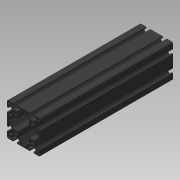
# Autodesk Inventor part: 3030-LS
Saved by Autodesk Inventor 2013 (Build 170138000, 138)
## iProperties
Company: 80/20 Inc.
Created: 2014-04-23
Part Number: 3030-LS
Material: Generic
Document SubType Name: Modeling
Density: 1 g/cm^3
Vendor: 80/20 Inc.
Engineer: Ross Bowman
Designer: Ross Bowman
Catalog Web Link: 8020.net
Material: 6105-T5 Aluminum
Author: Ross Bowman
Keywords: 80/20 , 8020 , T-Slot , Extrusion
Autodesk Inventor part; units mm, degrees
ref_plane "YZ Plane" through (0, 0, 0) normal (1, 0, 0) x (0, 1, 0)
ref_plane "XZ Plane" through (0, 0, 0) normal (0, 1, 0) x (-1, 0, 0)
ref_plane "XY Plane" through (0, 0, 0) normal (0, 0, 1) x (1, 0, 0)
sketch "Sketch1" plane through (0, 0, 0) normal (0, 0, 1) x (1, 0, 0)
  arc A0 (14.8044, -21.6898) -> (16.4102, -23.2956) centre (15.5149, -22.5851) ccw
  line L0 (16.0771, -20.4064) -> (14.8044, -21.6898)
  arc A1 (16.0771, -17.6936) -> (16.0771, -20.4064) centre (19.05, -19.05) ccw
  line L1 (14.7067, -16.3231) -> (16.0771, -17.6936)
  arc A2 (16.3231, -14.7067) -> (14.7067, -16.3231) centre (15.5149, -15.5149) ccw
  line L2 (17.6936, -16.0771) -> (16.3231, -14.7067)
  arc A3 (20.4064, -16.0771) -> (17.6936, -16.0771) centre (19.05, -19.05) ccw
  line L3 (21.7769, -14.7067) -> (20.4064, -16.0771)
  arc A4 (23.3933, -16.3231) -> (21.7769, -14.7067) centre (22.5851, -15.5149) ccw
  line L4 (22.0229, -17.6936) -> (23.3933, -16.3231)
  arc A5 (22.0229, -20.4064) -> (22.0229, -17.6936) centre (19.05, -19.05) ccw
  line L5 (23.3933, -21.7769) -> (22.0229, -20.4064)
  arc A6 (21.7769, -23.3933) -> (23.3933, -21.7769) centre (22.5851, -22.5851) ccw
  line L6 (20.4064, -22.0229) -> (21.7769, -23.3933)
  arc A7 (17.6936, -22.0229) -> (20.4064, -22.0229) centre (19.05, -19.05) ccw
  line L7 (16.4102, -23.2956) -> (17.6936, -22.0229)
  arc A8 (30.9118, -35.9156) -> (31.2928, -36.2966) centre (31.2928, -35.9156) ccw
  line L8 (30.9118, -31.2928) -> (30.9118, -35.9156)
  arc A9 (31.2928, -30.9118) -> (30.9118, -31.2928) centre (31.2928, -31.2928) ccw
  line L9 (35.9156, -30.9118) -> (31.2928, -30.9118)
  arc A10 (36.2966, -31.2928) -> (35.9156, -30.9118) centre (35.9156, -31.2928) ccw
  line L10 (36.2966, -33.5026) -> (36.2966, -31.2928)
  arc A11 (33.5026, -36.2966) -> (36.2966, -33.5026) centre (33.5026, -33.5026) ccw
  line L11 (31.2928, -36.2966) -> (33.5026, -36.2966)
  arc A12 (33.8793, -2.0655) -> (33.8793, 2.0655) centre (31.8138, 0) ccw
  line L12 (25.0169, -10.9278) -> (33.8793, -2.0655)
  arc A13 (21.6583, -12.319) -> (25.0169, -10.9278) centre (21.6583, -7.5692) ccw
  line L13 (15.494, -12.319) -> (21.6583, -12.319)
  arc A14 (15.494, -12.319) -> (12.319, -15.494) centre (15.494, -15.494) ccw
  line L14 (12.319, -21.6583) -> (12.319, -15.494)
  arc A15 (10.9278, -25.0169) -> (12.319, -21.6583) centre (7.5692, -21.6583) ccw
  line L15 (2.0655, -33.8793) -> (10.9278, -25.0169)
  arc A16 (-2.0655, -33.8793) -> (2.0655, -33.8793) centre (0, -31.8138) ccw
  line L16 (-10.9278, -25.0169) -> (-2.0655, -33.8793)
  arc A17 (-12.319, -21.6583) -> (-10.9278, -25.0169) centre (-7.5692, -21.6583) ccw
  line L17 (-12.319, -15.494) -> (-12.319, -21.6583)
  arc A18 (-12.319, -15.494) -> (-15.494, -12.319) centre (-15.494, -15.494) ccw
  line L18 (-21.6583, -12.319) -> (-15.494, -12.319)
  arc A19 (-25.0169, -10.9278) -> (-21.6583, -12.319) centre (-21.6583, -7.5692) ccw
  line L19 (-33.8793, -2.0655) -> (-25.0169, -10.9278)
  arc A20 (-33.8793, 2.0655) -> (-33.8793, -2.0655) centre (-31.8138, 0) ccw
  line L20 (-25.0169, 10.9278) -> (-33.8793, 2.0655)
  arc A21 (-21.6583, 12.319) -> (-25.0169, 10.9278) centre (-21.6583, 7.5692) ccw
  line L21 (-15.494, 12.319) -> (-21.6583, 12.319)
  arc A22 (-15.494, 12.319) -> (-12.319, 15.494) centre (-15.494, 15.494) ccw
  line L22 (-12.319, 21.6583) -> (-12.319, 15.494)
  arc A23 (-10.9278, 25.0169) -> (-12.319, 21.6583) centre (-7.5692, 21.6583) ccw
  line L23 (-2.0655, 33.8793) -> (-10.9278, 25.0169)
  arc A24 (2.0655, 33.8793) -> (-2.0655, 33.8793) centre (0, 31.8138) ccw
  line L24 (10.9278, 25.0169) -> (2.0655, 33.8793)
  arc A25 (12.319, 21.6583) -> (10.9278, 25.0169) centre (7.5692, 21.6583) ccw
  line L25 (12.319, 15.494) -> (12.319, 21.6583)
  arc A26 (12.319, 15.494) -> (15.494, 12.319) centre (15.494, 15.494) ccw
  line L26 (21.6583, 12.319) -> (15.494, 12.319)
  arc A27 (25.0169, 10.9278) -> (21.6583, 12.319) centre (21.6583, 7.5692) ccw
  line L27 (33.8793, 2.0655) -> (25.0169, 10.9278)
  arc A28 (-16.4102, -23.2956) -> (-14.8044, -21.6898) centre (-15.5149, -22.5851) ccw
  line L28 (-17.6936, -22.0229) -> (-16.4102, -23.2956)
  arc A29 (-20.4064, -22.0229) -> (-17.6936, -22.0229) centre (-19.05, -19.05) ccw
  line L29 (-21.7769, -23.3933) -> (-20.4064, -22.0229)
  arc A30 (-23.3933, -21.7769) -> (-21.7769, -23.3933) centre (-22.5851, -22.5851) ccw
  line L30 (-22.0229, -20.4064) -> (-23.3933, -21.7769)
  arc A31 (-22.0229, -17.6936) -> (-22.0229, -20.4064) centre (-19.05, -19.05) ccw
  line L31 (-23.3933, -16.3231) -> (-22.0229, -17.6936)
  arc A32 (-21.7769, -14.7067) -> (-23.3933, -16.3231) centre (-22.5851, -15.5149) ccw
  line L32 (-20.4064, -16.0771) -> (-21.7769, -14.7067)
  arc A33 (-17.6936, -16.0771) -> (-20.4064, -16.0771) centre (-19.05, -19.05) ccw
  line L33 (-16.3231, -14.7067) -> (-17.6936, -16.0771)
  arc A34 (-14.7067, -16.3231) -> (-16.3231, -14.7067) centre (-15.5149, -15.5149) ccw
  line L34 (-16.0771, -17.6936) -> (-14.7067, -16.3231)
  arc A35 (-16.0771, -20.4064) -> (-16.0771, -17.6936) centre (-19.05, -19.05) ccw
  line L35 (-14.8044, -21.6898) -> (-16.0771, -20.4064)
  arc A36 (-31.2928, -36.2966) -> (-30.9118, -35.9156) centre (-31.2928, -35.9156) ccw
  line L36 (-33.5026, -36.2966) -> (-31.2928, -36.2966)
  arc A37 (-36.2966, -33.5026) -> (-33.5026, -36.2966) centre (-33.5026, -33.5026) ccw
  line L37 (-36.2966, -31.2928) -> (-36.2966, -33.5026)
  arc A38 (-35.9156, -30.9118) -> (-36.2966, -31.2928) centre (-35.9156, -31.2928) ccw
  line L38 (-31.2928, -30.9118) -> (-35.9156, -30.9118)
  arc A39 (-30.9118, -31.2928) -> (-31.2928, -30.9118) centre (-31.2928, -31.2928) ccw
  line L39 (-30.9118, -35.9156) -> (-30.9118, -31.2928)
  arc A40 (16.4102, 23.2956) -> (14.8044, 21.6898) centre (15.5149, 22.5851) ccw
  line L40 (17.6936, 22.0229) -> (16.4102, 23.2956)
  arc A41 (20.4064, 22.0229) -> (17.6936, 22.0229) centre (19.05, 19.05) ccw
  line L41 (21.7769, 23.3933) -> (20.4064, 22.0229)
  arc A42 (23.3933, 21.7769) -> (21.7769, 23.3933) centre (22.5851, 22.5851) ccw
  line L42 (22.0229, 20.4064) -> (23.3933, 21.7769)
  arc A43 (22.0229, 17.6936) -> (22.0229, 20.4064) centre (19.05, 19.05) ccw
  line L43 (23.3933, 16.3231) -> (22.0229, 17.6936)
  arc A44 (21.7769, 14.7067) -> (23.3933, 16.3231) centre (22.5851, 15.5149) ccw
  line L44 (20.4064, 16.0771) -> (21.7769, 14.7067)
  arc A45 (17.6936, 16.0771) -> (20.4064, 16.0771) centre (19.05, 19.05) ccw
  line L45 (16.3231, 14.7067) -> (17.6936, 16.0771)
  arc A46 (14.7067, 16.3231) -> (16.3231, 14.7067) centre (15.5149, 15.5149) ccw
  line L46 (16.0771, 17.6936) -> (14.7067, 16.3231)
  arc A47 (16.0771, 20.4064) -> (16.0771, 17.6936) centre (19.05, 19.05) ccw
  line L47 (14.8044, 21.6898) -> (16.0771, 20.4064)
  arc A48 (31.2928, 36.2966) -> (30.9118, 35.9156) centre (31.2928, 35.9156) ccw
  line L48 (33.5026, 36.2966) -> (31.2928, 36.2966)
  arc A49 (36.2966, 33.5026) -> (33.5026, 36.2966) centre (33.5026, 33.5026) ccw
  line L49 (36.2966, 31.2928) -> (36.2966, 33.5026)
  arc A50 (35.9156, 30.9118) -> (36.2966, 31.2928) centre (35.9156, 31.2928) ccw
  line L50 (31.2928, 30.9118) -> (35.9156, 30.9118)
  arc A51 (30.9118, 31.2928) -> (31.2928, 30.9118) centre (31.2928, 31.2928) ccw
  line L51 (30.9118, 35.9156) -> (30.9118, 31.2928)
  arc A52 (-14.8044, 21.6898) -> (-16.4102, 23.2956) centre (-15.5149, 22.5851) ccw
  line L52 (-16.0771, 20.4064) -> (-14.8044, 21.6898)
  arc A53 (-16.0771, 17.6936) -> (-16.0771, 20.4064) centre (-19.05, 19.05) ccw
  line L53 (-14.7067, 16.3231) -> (-16.0771, 17.6936)
  arc A54 (-16.3231, 14.7067) -> (-14.7067, 16.3231) centre (-15.5149, 15.5149) ccw
  line L54 (-17.6936, 16.0771) -> (-16.3231, 14.7067)
  arc A55 (-20.4064, 16.0771) -> (-17.6936, 16.0771) centre (-19.05, 19.05) ccw
  line L55 (-21.7769, 14.7067) -> (-20.4064, 16.0771)
  arc A56 (-23.3933, 16.3231) -> (-21.7769, 14.7067) centre (-22.5851, 15.5149) ccw
  line L56 (-22.0229, 17.6936) -> (-23.3933, 16.3231)
  arc A57 (-22.0229, 20.4064) -> (-22.0229, 17.6936) centre (-19.05, 19.05) ccw
  line L57 (-23.3933, 21.7769) -> (-22.0229, 20.4064)
  arc A58 (-21.7769, 23.3933) -> (-23.3933, 21.7769) centre (-22.5851, 22.5851) ccw
  line L58 (-20.4064, 22.0229) -> (-21.7769, 23.3933)
  arc A59 (-17.6936, 22.0229) -> (-20.4064, 22.0229) centre (-19.05, 19.05) ccw
  line L59 (-16.4102, 23.2956) -> (-17.6936, 22.0229)
  arc A60 (-30.9118, 35.9156) -> (-31.2928, 36.2966) centre (-31.2928, 35.9156) ccw
  line L60 (-30.9118, 31.2928) -> (-30.9118, 35.9156)
  arc A61 (-31.2928, 30.9118) -> (-30.9118, 31.2928) centre (-31.2928, 31.2928) ccw
  line L61 (-35.9156, 30.9118) -> (-31.2928, 30.9118)
  arc A62 (-36.2966, 31.2928) -> (-35.9156, 30.9118) centre (-35.9156, 31.2928) ccw
  line L62 (-36.2966, 33.5026) -> (-36.2966, 31.2928)
  arc A63 (-33.5026, 36.2966) -> (-36.2966, 33.5026) centre (-33.5026, 33.5026) ccw
  line L63 (-31.2928, 36.2966) -> (-33.5026, 36.2966)
  arc A64 (34.8742, -26.289) -> (34.4932, -25.908) centre (34.4932, -26.289) ccw
  line L64 (34.8742, -26.289) -> (34.8742, -28.063)
  arc A65 (33.6042, -29.337) -> (34.8742, -28.063) centre (33.6042, -28.067) ccw
  line L65 (33.6042, -29.337) -> (32.0183, -29.337)
  arc A66 (31.1203, -28.965) -> (32.0183, -29.337) centre (32.0183, -28.067) ccw
  line L66 (31.1203, -28.965) -> (27.1722, -25.0169)
  arc A67 (25.781, -21.6583) -> (27.1722, -25.0169) centre (30.5308, -21.6583) ccw
  line L67 (25.781, -21.6583) -> (25.781, -16.4417)
  arc A68 (27.1722, -13.0831) -> (25.781, -16.4417) centre (30.5308, -16.4417) ccw
  line L68 (27.1722, -13.0831) -> (31.1203, -9.135)
  arc A69 (32.0183, -8.763) -> (31.1203, -9.135) centre (32.0183, -10.033) ccw
  line L69 (32.0183, -8.763) -> (33.6042, -8.763)
  arc A70 (34.8742, -10.037) -> (33.6042, -8.763) centre (33.6042, -10.033) ccw
  line L70 (34.8742, -10.037) -> (34.8742, -11.811)
  arc A71 (34.4932, -12.192) -> (34.8742, -11.811) centre (34.4932, -11.811) ccw
  line L71 (34.4932, -12.192) -> (34.417, -12.192)
  arc A72 (34.417, -12.192) -> (34.036, -12.573) centre (34.417, -12.573) ccw
  line L72 (34.036, -12.573) -> (34.036, -13.4112)
  arc A73 (34.036, -13.4112) -> (35.6108, -14.986) centre (35.6108, -13.4112) ccw
  line L73 (35.6108, -14.986) -> (36.5252, -14.986)
  arc A74 (36.5252, -14.986) -> (38.1, -13.4112) centre (36.5252, -13.4112) ccw
  line L74 (38.1, -13.4112) -> (38.1, 13.4112)
  arc A75 (38.1, 13.4112) -> (36.5252, 14.986) centre (36.5252, 13.4112) ccw
  line L75 (36.5252, 14.986) -> (35.6108, 14.986)
  arc A76 (35.6108, 14.986) -> (34.036, 13.4112) centre (35.6108, 13.4112) ccw
  line L76 (34.036, 13.4112) -> (34.036, 12.573)
  arc A77 (34.036, 12.573) -> (34.417, 12.192) centre (34.417, 12.573) ccw
  line L77 (34.417, 12.192) -> (34.4932, 12.192)
  arc A78 (34.8742, 11.811) -> (34.4932, 12.192) centre (34.4932, 11.811) ccw
  line L78 (34.8742, 11.811) -> (34.8742, 10.037)
  arc A79 (33.6042, 8.763) -> (34.8742, 10.037) centre (33.6042, 10.033) ccw
  line L79 (33.6042, 8.763) -> (32.0183, 8.763)
  arc A80 (31.1203, 9.135) -> (32.0183, 8.763) centre (32.0183, 10.033) ccw
  line L80 (31.1203, 9.135) -> (27.1722, 13.0831)
  arc A81 (25.781, 16.4417) -> (27.1722, 13.0831) centre (30.5308, 16.4417) ccw
  line L81 (25.781, 16.4417) -> (25.781, 21.6583)
  arc A82 (27.1722, 25.0169) -> (25.781, 21.6583) centre (30.5308, 21.6583) ccw
  line L82 (27.1722, 25.0169) -> (31.1203, 28.965)
  arc A83 (32.0183, 29.337) -> (31.1203, 28.965) centre (32.0183, 28.067) ccw
  line L83 (32.0183, 29.337) -> (33.6042, 29.337)
  arc A84 (34.8742, 28.063) -> (33.6042, 29.337) centre (33.6042, 28.067) ccw
  line L84 (34.8742, 28.063) -> (34.8742, 26.289)
  arc A85 (34.4932, 25.908) -> (34.8742, 26.289) centre (34.4932, 26.289) ccw
  line L85 (34.4932, 25.908) -> (34.417, 25.908)
  arc A86 (34.417, 25.908) -> (34.036, 25.527) centre (34.417, 25.527) ccw
  line L86 (34.036, 25.527) -> (34.036, 24.6888)
  arc A87 (34.036, 24.6888) -> (35.6108, 23.114) centre (35.6108, 24.6888) ccw
  line L87 (35.6108, 23.114) -> (36.5252, 23.114)
  arc A88 (36.5252, 23.114) -> (38.1, 24.6888) centre (36.5252, 24.6888) ccw
  line L88 (38.1, 24.6888) -> (38.1, 34.925)
  arc A89 (38.1, 34.925) -> (34.925, 38.1) centre (34.925, 34.925) ccw
  line L89 (34.925, 38.1) -> (24.6888, 38.1)
  arc A90 (24.6888, 38.1) -> (23.114, 36.5252) centre (24.6888, 36.5252) ccw
  line L90 (23.114, 36.5252) -> (23.114, 35.6108)
  arc A91 (23.114, 35.6108) -> (24.6888, 34.036) centre (24.6888, 35.6108) ccw
  line L91 (24.6888, 34.036) -> (25.527, 34.036)
  arc A92 (25.527, 34.036) -> (25.908, 34.417) centre (25.527, 34.417) ccw
  line L92 (25.908, 34.417) -> (25.908, 34.4932)
  arc A93 (26.289, 34.8742) -> (25.908, 34.4932) centre (26.289, 34.4932) ccw
  line L93 (26.289, 34.8742) -> (28.063, 34.8742)
  arc A94 (29.337, 33.6042) -> (28.063, 34.8742) centre (28.067, 33.6042) ccw
  line L94 (29.337, 33.6042) -> (29.337, 32.0183)
  arc A95 (28.965, 31.1203) -> (29.337, 32.0183) centre (28.067, 32.0183) ccw
  line L95 (28.965, 31.1203) -> (25.0169, 27.1722)
  arc A96 (21.6583, 25.781) -> (25.0169, 27.1722) centre (21.6583, 30.5308) ccw
  line L96 (21.6583, 25.781) -> (16.4417, 25.781)
  arc A97 (13.0831, 27.1722) -> (16.4417, 25.781) centre (16.4417, 30.5308) ccw
  line L97 (13.0831, 27.1722) -> (9.135, 31.1203)
  arc A98 (8.763, 32.0183) -> (9.135, 31.1203) centre (10.033, 32.0183) ccw
  line L98 (8.763, 32.0183) -> (8.763, 33.6042)
  arc A99 (10.037, 34.8742) -> (8.763, 33.6042) centre (10.033, 33.6042) ccw
  line L99 (10.037, 34.8742) -> (11.811, 34.8742)
  arc A100 (12.192, 34.4932) -> (11.811, 34.8742) centre (11.811, 34.4932) ccw
  line L100 (12.192, 34.4932) -> (12.192, 34.417)
  arc A101 (12.192, 34.417) -> (12.573, 34.036) centre (12.573, 34.417) ccw
  line L101 (12.573, 34.036) -> (13.4112, 34.036)
  arc A102 (13.4112, 34.036) -> (14.986, 35.6108) centre (13.4112, 35.6108) ccw
  line L102 (14.986, 35.6108) -> (14.986, 36.5252)
  arc A103 (14.986, 36.5252) -> (13.4112, 38.1) centre (13.4112, 36.5252) ccw
  line L103 (13.4112, 38.1) -> (-13.4112, 38.1)
  arc A104 (-13.4112, 38.1) -> (-14.986, 36.5252) centre (-13.4112, 36.5252) ccw
  line L104 (-14.986, 36.5252) -> (-14.986, 35.6108)
  arc A105 (-14.986, 35.6108) -> (-13.4112, 34.036) centre (-13.4112, 35.6108) ccw
  line L105 (-13.4112, 34.036) -> (-12.573, 34.036)
  arc A106 (-12.573, 34.036) -> (-12.192, 34.417) centre (-12.573, 34.417) ccw
  line L106 (-12.192, 34.417) -> (-12.192, 34.4932)
  arc A107 (-11.811, 34.8742) -> (-12.192, 34.4932) centre (-11.811, 34.4932) ccw
  line L107 (-11.811, 34.8742) -> (-10.037, 34.8742)
  arc A108 (-8.763, 33.6042) -> (-10.037, 34.8742) centre (-10.033, 33.6042) ccw
  line L108 (-8.763, 33.6042) -> (-8.763, 32.0183)
  arc A109 (-9.135, 31.1203) -> (-8.763, 32.0183) centre (-10.033, 32.0183) ccw
  line L109 (-9.135, 31.1203) -> (-13.0831, 27.1722)
  arc A110 (-16.4417, 25.781) -> (-13.0831, 27.1722) centre (-16.4417, 30.5308) ccw
  line L110 (-16.4417, 25.781) -> (-21.6583, 25.781)
  arc A111 (-25.0169, 27.1722) -> (-21.6583, 25.781) centre (-21.6583, 30.5308) ccw
  line L111 (-25.0169, 27.1722) -> (-28.965, 31.1203)
  arc A112 (-29.337, 32.0183) -> (-28.965, 31.1203) centre (-28.067, 32.0183) ccw
  line L112 (-29.337, 32.0183) -> (-29.337, 33.6042)
  arc A113 (-28.063, 34.8742) -> (-29.337, 33.6042) centre (-28.067, 33.6042) ccw
  line L113 (-28.063, 34.8742) -> (-26.289, 34.8742)
  arc A114 (-25.908, 34.4932) -> (-26.289, 34.8742) centre (-26.289, 34.4932) ccw
  line L114 (-25.908, 34.4932) -> (-25.908, 34.417)
  arc A115 (-25.908, 34.417) -> (-25.527, 34.036) centre (-25.527, 34.417) ccw
  line L115 (-25.527, 34.036) -> (-24.6888, 34.036)
  arc A116 (-24.6888, 34.036) -> (-23.114, 35.6108) centre (-24.6888, 35.6108) ccw
  line L116 (-23.114, 35.6108) -> (-23.114, 36.5252)
  arc A117 (-23.114, 36.5252) -> (-24.6888, 38.1) centre (-24.6888, 36.5252) ccw
  line L117 (-24.6888, 38.1) -> (-34.925, 38.1)
  arc A118 (-34.925, 38.1) -> (-38.1, 34.925) centre (-34.925, 34.925) ccw
  line L118 (-38.1, 34.925) -> (-38.1, 24.6888)
  arc A119 (-38.1, 24.6888) -> (-36.5252, 23.114) centre (-36.5252, 24.6888) ccw
  line L119 (-36.5252, 23.114) -> (-35.6108, 23.114)
  arc A120 (-35.6108, 23.114) -> (-34.036, 24.6888) centre (-35.6108, 24.6888) ccw
  line L120 (-34.036, 24.6888) -> (-34.036, 25.527)
  arc A121 (-34.036, 25.527) -> (-34.417, 25.908) centre (-34.417, 25.527) ccw
  line L121 (-34.417, 25.908) -> (-34.4932, 25.908)
  arc A122 (-34.8742, 26.289) -> (-34.4932, 25.908) centre (-34.4932, 26.289) ccw
  line L122 (-34.8742, 26.289) -> (-34.8742, 28.063)
  arc A123 (-33.6042, 29.337) -> (-34.8742, 28.063) centre (-33.6042, 28.067) ccw
  line L123 (-33.6042, 29.337) -> (-32.0183, 29.337)
  arc A124 (-31.1203, 28.965) -> (-32.0183, 29.337) centre (-32.0183, 28.067) ccw
  line L124 (-31.1203, 28.965) -> (-27.1722, 25.0169)
  arc A125 (-25.781, 21.6583) -> (-27.1722, 25.0169) centre (-30.5308, 21.6583) ccw
  line L125 (-25.781, 21.6583) -> (-25.781, 16.4417)
  arc A126 (-27.1722, 13.0831) -> (-25.781, 16.4417) centre (-30.5308, 16.4417) ccw
  line L126 (-27.1722, 13.0831) -> (-31.1203, 9.135)
  arc A127 (-32.0183, 8.763) -> (-31.1203, 9.135) centre (-32.0183, 10.033) ccw
  line L127 (-32.0183, 8.763) -> (-33.6042, 8.763)
  arc A128 (-34.8742, 10.037) -> (-33.6042, 8.763) centre (-33.6042, 10.033) ccw
  line L128 (-34.8742, 10.037) -> (-34.8742, 11.811)
  arc A129 (-34.4932, 12.192) -> (-34.8742, 11.811) centre (-34.4932, 11.811) ccw
  line L129 (-34.4932, 12.192) -> (-34.417, 12.192)
  arc A130 (-34.417, 12.192) -> (-34.036, 12.573) centre (-34.417, 12.573) ccw
  line L130 (-34.036, 12.573) -> (-34.036, 13.4112)
  arc A131 (-34.036, 13.4112) -> (-35.6108, 14.986) centre (-35.6108, 13.4112) ccw
  line L131 (-35.6108, 14.986) -> (-36.5252, 14.986)
  arc A132 (-36.5252, 14.986) -> (-38.1, 13.4112) centre (-36.5252, 13.4112) ccw
  line L132 (-38.1, 13.4112) -> (-38.1, -13.4112)
  arc A133 (-38.1, -13.4112) -> (-36.5252, -14.986) centre (-36.5252, -13.4112) ccw
  line L133 (-36.5252, -14.986) -> (-35.6108, -14.986)
  arc A134 (-35.6108, -14.986) -> (-34.036, -13.4112) centre (-35.6108, -13.4112) ccw
  line L134 (-34.036, -13.4112) -> (-34.036, -12.573)
  arc A135 (-34.036, -12.573) -> (-34.417, -12.192) centre (-34.417, -12.573) ccw
  line L135 (-34.417, -12.192) -> (-34.4932, -12.192)
  arc A136 (-34.8742, -11.811) -> (-34.4932, -12.192) centre (-34.4932, -11.811) ccw
  line L136 (-34.8742, -11.811) -> (-34.8742, -10.037)
  arc A137 (-33.6042, -8.763) -> (-34.8742, -10.037) centre (-33.6042, -10.033) ccw
  line L137 (-33.6042, -8.763) -> (-32.0183, -8.763)
  arc A138 (-31.1203, -9.135) -> (-32.0183, -8.763) centre (-32.0183, -10.033) ccw
  line L138 (-31.1203, -9.135) -> (-27.1722, -13.0831)
  arc A139 (-25.781, -16.4417) -> (-27.1722, -13.0831) centre (-30.5308, -16.4417) ccw
  line L139 (-25.781, -16.4417) -> (-25.781, -21.6583)
  arc A140 (-27.1722, -25.0169) -> (-25.781, -21.6583) centre (-30.5308, -21.6583) ccw
  line L140 (-27.1722, -25.0169) -> (-31.1203, -28.965)
  arc A141 (-32.0183, -29.337) -> (-31.1203, -28.965) centre (-32.0183, -28.067) ccw
  line L141 (-32.0183, -29.337) -> (-33.6042, -29.337)
  arc A142 (-34.8742, -28.063) -> (-33.6042, -29.337) centre (-33.6042, -28.067) ccw
  line L142 (-34.8742, -28.063) -> (-34.8742, -26.289)
  arc A143 (-34.4932, -25.908) -> (-34.8742, -26.289) centre (-34.4932, -26.289) ccw
  line L143 (-34.4932, -25.908) -> (-34.417, -25.908)
  arc A144 (-34.417, -25.908) -> (-34.036, -25.527) centre (-34.417, -25.527) ccw
  line L144 (-34.036, -25.527) -> (-34.036, -24.6888)
  arc A145 (-34.036, -24.6888) -> (-35.6108, -23.114) centre (-35.6108, -24.6888) ccw
  line L145 (-35.6108, -23.114) -> (-36.5252, -23.114)
  arc A146 (-36.5252, -23.114) -> (-38.1, -24.6888) centre (-36.5252, -24.6888) ccw
  line L146 (-38.1, -24.6888) -> (-38.1, -34.925)
  arc A147 (-38.1, -34.925) -> (-34.925, -38.1) centre (-34.925, -34.925) ccw
  line L147 (-34.925, -38.1) -> (-24.6888, -38.1)
  arc A148 (-24.6888, -38.1) -> (-23.114, -36.5252) centre (-24.6888, -36.5252) ccw
  line L148 (-23.114, -36.5252) -> (-23.114, -35.6108)
  arc A149 (-23.114, -35.6108) -> (-24.6888, -34.036) centre (-24.6888, -35.6108) ccw
  line L149 (-24.6888, -34.036) -> (-25.527, -34.036)
  arc A150 (-25.527, -34.036) -> (-25.908, -34.417) centre (-25.527, -34.417) ccw
  line L150 (-25.908, -34.417) -> (-25.908, -34.4932)
  arc A151 (-26.289, -34.8742) -> (-25.908, -34.4932) centre (-26.289, -34.4932) ccw
  line L151 (-26.289, -34.8742) -> (-28.063, -34.8742)
  arc A152 (-29.337, -33.6042) -> (-28.063, -34.8742) centre (-28.067, -33.6042) ccw
  line L152 (-29.337, -33.6042) -> (-29.337, -32.0183)
  arc A153 (-28.965, -31.1203) -> (-29.337, -32.0183) centre (-28.067, -32.0183) ccw
  line L153 (-28.965, -31.1203) -> (-25.0169, -27.1722)
  arc A154 (-21.6583, -25.781) -> (-25.0169, -27.1722) centre (-21.6583, -30.5308) ccw
  line L154 (-21.6583, -25.781) -> (-16.4417, -25.781)
  arc A155 (-13.0831, -27.1722) -> (-16.4417, -25.781) centre (-16.4417, -30.5308) ccw
  line L155 (-13.0831, -27.1722) -> (-9.135, -31.1203)
  arc A156 (-8.763, -32.0183) -> (-9.135, -31.1203) centre (-10.033, -32.0183) ccw
  line L156 (-8.763, -32.0183) -> (-8.763, -33.6042)
  arc A157 (-10.037, -34.8742) -> (-8.763, -33.6042) centre (-10.033, -33.6042) ccw
  line L157 (-10.037, -34.8742) -> (-11.811, -34.8742)
  arc A158 (-12.192, -34.4932) -> (-11.811, -34.8742) centre (-11.811, -34.4932) ccw
  line L158 (-12.192, -34.4932) -> (-12.192, -34.417)
  arc A159 (-12.192, -34.417) -> (-12.573, -34.036) centre (-12.573, -34.417) ccw
  line L159 (-12.573, -34.036) -> (-13.4112, -34.036)
  arc A160 (-13.4112, -34.036) -> (-14.986, -35.6108) centre (-13.4112, -35.6108) ccw
  line L160 (-14.986, -35.6108) -> (-14.986, -36.5252)
  arc A161 (-14.986, -36.5252) -> (-13.4112, -38.1) centre (-13.4112, -36.5252) ccw
  line L161 (-13.4112, -38.1) -> (13.4112, -38.1)
  arc A162 (13.4112, -38.1) -> (14.986, -36.5252) centre (13.4112, -36.5252) ccw
  line L162 (14.986, -36.5252) -> (14.986, -35.6108)
  arc A163 (14.986, -35.6108) -> (13.4112, -34.036) centre (13.4112, -35.6108) ccw
  line L163 (13.4112, -34.036) -> (12.573, -34.036)
  arc A164 (12.573, -34.036) -> (12.192, -34.417) centre (12.573, -34.417) ccw
  line L164 (12.192, -34.417) -> (12.192, -34.4932)
  arc A165 (11.811, -34.8742) -> (12.192, -34.4932) centre (11.811, -34.4932) ccw
  line L165 (11.811, -34.8742) -> (10.037, -34.8742)
  arc A166 (8.763, -33.6042) -> (10.037, -34.8742) centre (10.033, -33.6042) ccw
  line L166 (8.763, -33.6042) -> (8.763, -32.0183)
  arc A167 (9.135, -31.1203) -> (8.763, -32.0183) centre (10.033, -32.0183) ccw
  line L167 (9.135, -31.1203) -> (13.0831, -27.1722)
  arc A168 (16.4417, -25.781) -> (13.0831, -27.1722) centre (16.4417, -30.5308) ccw
  line L168 (16.4417, -25.781) -> (21.6583, -25.781)
  arc A169 (25.0169, -27.1722) -> (21.6583, -25.781) centre (21.6583, -30.5308) ccw
  line L169 (25.0169, -27.1722) -> (28.965, -31.1203)
  arc A170 (29.337, -32.0183) -> (28.965, -31.1203) centre (28.067, -32.0183) ccw
  line L170 (29.337, -32.0183) -> (29.337, -33.6042)
  arc A171 (28.063, -34.8742) -> (29.337, -33.6042) centre (28.067, -33.6042) ccw
  line L171 (28.063, -34.8742) -> (26.289, -34.8742)
  arc A172 (25.908, -34.4932) -> (26.289, -34.8742) centre (26.289, -34.4932) ccw
  line L172 (25.908, -34.4932) -> (25.908, -34.417)
  arc A173 (25.908, -34.417) -> (25.527, -34.036) centre (25.527, -34.417) ccw
  line L173 (25.527, -34.036) -> (24.6888, -34.036)
  arc A174 (24.6888, -34.036) -> (23.114, -35.6108) centre (24.6888, -35.6108) ccw
  line L174 (23.114, -35.6108) -> (23.114, -36.5252)
  arc A175 (23.114, -36.5252) -> (24.6888, -38.1) centre (24.6888, -36.5252) ccw
  line L175 (24.6888, -38.1) -> (34.925, -38.1)
  arc A176 (34.925, -38.1) -> (38.1, -34.925) centre (34.925, -34.925) ccw
  line L176 (38.1, -34.925) -> (38.1, -24.6888)
  arc A177 (38.1, -24.6888) -> (36.5252, -23.114) centre (36.5252, -24.6888) ccw
  line L177 (36.5252, -23.114) -> (35.6108, -23.114)
  arc A178 (35.6108, -23.114) -> (34.036, -24.6888) centre (35.6108, -24.6888) ccw
  line L178 (34.036, -24.6888) -> (34.036, -25.527)
  arc A179 (34.036, -25.527) -> (34.417, -25.908) centre (34.417, -25.527) ccw
  line L179 (34.417, -25.908) -> (34.4932, -25.908)
  point P0 (0, 0)
  constraints: 360 end point, 360 point on circle, 180 centre point
extrude "Extrusion1" add sketch "Sketch1" against normal blind 304.8
body "Solid1"
